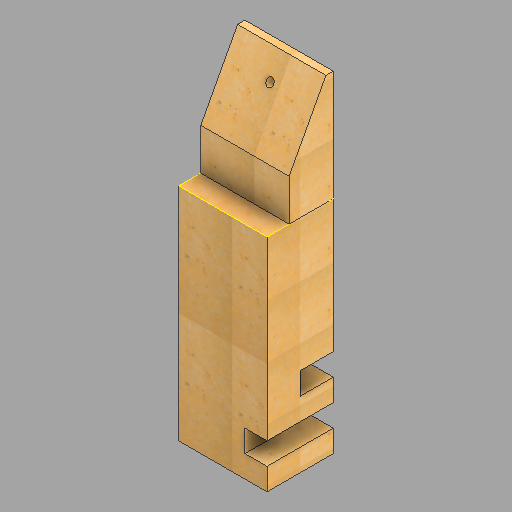
# Autodesk Inventor part: blocks
Saved by Autodesk Inventor 2023 (Build 270158030, 158C)
## iProperties
RuleStatus: InUse
Created: 2022-06-24
Part Number: blocks
Material: Granite, Cut, Polished
Document SubType Name: Modeling
Designer: awelt
Mass: 1.10864e+07 g
Surface Area: 220655 cm^2
Volume: 4.10608e+06 cm^3
Density: 2.7 g/cm^3
Appearance: Amber Select
AfterDocSave0: Convert in3 volume to ft3
in3 to ft3: 0.08
TEST: 0.084
Author: awelt
Autodesk Inventor part; units mm, degrees
ref_plane "YZ Plane" through (0, 0, 0) normal (1, 0, 0) x (0, 1, 0)
ref_plane "XZ Plane" through (0, 0, 0) normal (0, 1, 0) x (-1, 0, 0)
ref_plane "XY Plane" through (0, 0, 0) normal (0, 0, 1) x (1, 0, 0)
sketch "Sketch1" plane through (0, 0, 0) normal (1, 0, 0) x (0, 1, 0)
  line L0 (0, 0) -> (4572, 0)
  line L1 (0, 0) -> (0, 914.4)
  line L2 (0, 914.4) -> (3048, 914.4)
  line L3 (3048, 914.4) -> (3048, 609.6)
  line L4 (4572, 0) -> (4572, 101.4984)
  line L5 (4572, 101.4984) -> (3619.4286, 609.6)
  line L6 (3048, 609.6) -> (3619.4286, 609.6)
  dimension "d0" = 4572
  dimension "d1" = 914.4
  dimension "d2" = 3048
  dimension "d3" = 304.8
  dimension "d4" = 101.4984
  dimension "d5" = 571.4286
  constraints: 14 end point, 3 perpendicular, 2 vertical, 1 horizontal
  measures "d0" distance of L0.start L0.end
  measures "d1" distance of L0.start L1.end
  measures "d2" distance of L1.end L2.end
  measures "d3" distance of L2.end L3.end
  measures "d4" distance of L0.end L4.end
  measures "d5" distance of L3.end L5.end
extrude "Extrusion1" add sketch "Sketch1" along normal blind 1219.2
sketch "Sketch2" plane through (1219.2, 0, 0) normal (1, 0, 0) x (0, 0, -1)
  line L0 (0, 0) -> (0, 4572) projected
  line L1 (-914.4, 3048) -> (-914.4, 0) projected
  line L2 (0, 609.6) -> (-914.4, 609.6)
  line L3 (-914.4, 609.6) -> (-914.4, 304.8)
  line L4 (-914.4, 304.8) -> (0, 304.8)
  line L5 (0, 304.8) -> (0, 609.6)
  line L6 (0, 1219.2) -> (-914.4, 1219.2)
  line L7 (-914.4, 1219.2) -> (-914.4, 914.4)
  line L8 (-914.4, 914.4) -> (0, 914.4)
  line L9 (0, 914.4) -> (0, 1219.2)
  line L10 (-457.2, 1219.2) -> (-457.2, 914.4)
  point P0 (0, 304.8)
  point P1 (0, 914.4)
  dimension "d8" = 304.8
  dimension "d9" = 304.8
  dimension "d10" = 304.8
  dimension "d11" = 304.8
  dimension "d12" = 304.8
  dimension "d13" = 304.8
  constraints: 18 end point, 6 point on line, 4 parallel, 2 horizontal, 2 midpoint, 2 perpendicular
  measures "d8" distance of point (0, 304.8) L0.start
  measures "d9" distance of L2.start point (0, 304.8)
  measures "d10" distance of point (0, 914.4) L2.start
  measures "d11" distance of L6.start point (0, 914.4)
  measures "d12" distance between parallel lines of L4 L2
  measures "d13" distance between parallel lines of L8 L6
extrude "Extrusion2" cut sketch "Sketch2" against normal blind 304.8 contours L4 L1 L2 L0 | L8 L10 L6 L0
sketch "Sketch3" plane through (0, 3048, 609.6) normal (0, 0, 1) x (1, 0, 0)
  line L0 (0, 1524) -> (0, 571.4286) projected
  line L1 (0, 571.4286) -> (1219.2, 571.4286) projected
  line L2 (1219.2, 1524) -> (1219.2, 571.4286) projected
  line L3 (0, 1524) -> (1219.2, 1524) projected
  line L4 (0, 1524) -> (1219.2, 1524) construction
  line L5 (609.6, 1524) -> (609.6, 571.4286) construction
  line L6 (0, -3048) -> (0, 1524) construction
  line L7 (0, 1219.2) -> (1219.2, 1219.2) construction
  circle A0 centre (609.6, 1219.2) radius 152.4 construction
  circle A1 centre (609.6, 1219.2) radius 50.8
  dimension "d16" = 304.8
  dimension "d17" = 304.8
  dimension "d18" = 101.6
  constraints: 4 end point, 3 midpoint, 2 centre point, 2 point on line, 1 coincident, 1 perpendicular
  measures "d16" distance between parallel lines of L3 L7
  measures "d17" diameter of A0
  measures "d18" diameter of A1
extrude "Extrusion3" cut sketch "Sketch3" against normal through all contours A1
sketch "Sketch5" plane through (1219.2, 0, 0) normal (1, 0, 0) x (0, 0, -1)
  line L0 (-1300.5956, 3048) -> (224.2837, 3048)
  point P0 (0, 0)
  point P1 (-914.4, 3048)
  constraints: 2 end point, 1 horizontal, 1 point on line
surface extrude "ExtrusionSrf1" sketch "Sketch5" against normal up to next shown yes curves L0
split body "Split1" result two bodies by surface "ExtrusionSrf1" first body at (711.2, 2235.2, 913.9)
equation "\"d9\" = d8"
equation "\"d10\" = d8"
body "Srf1"
